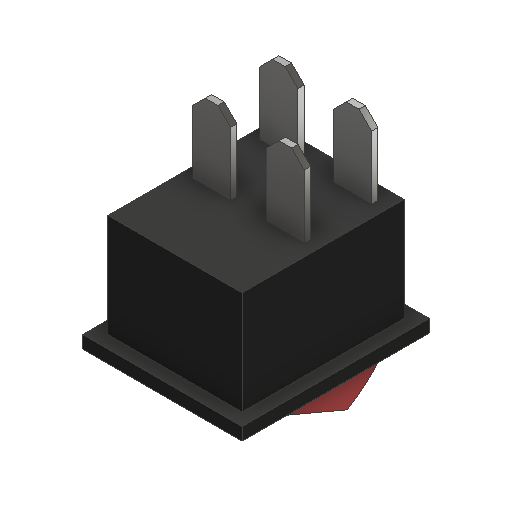
# Autodesk Inventor part: COTS_GENERIC_AC_Power_Switch_10A
Saved by Autodesk Inventor 2026.1 (Build 301233000, 233)
## iProperties
Created: 2016-06-24
Part Number: COTS_GENERIC_AC_Power_Switch_10A
Material: Ogólny
Document SubType Name: Modeling
Designer: Andrzej
Density: 1 g/cm^3
Appearance: Kauczuk - czarny
Mass: 12.2354 g
Surface Area: 41.2399 cm^2
Volume: 12.2354 cm^3
Author: Andrzej
Autodesk Inventor part; units mm, degrees
ref_plane "YZ Plane" through (0, 0, 0) normal (1, 0, 0) x (0, 1, 0)
ref_plane "XZ Plane" through (0, 0, 0) normal (0, 1, 0) x (-1, 0, 0)
sketch "Szkic1" plane through (0, 0, 0) normal (0, 0, 1) x (1, 0, 0)
  line L0 (-7.5735, 20.8135) -> (13.6265, 20.8135)
  line L1 (13.6265, 20.8135) -> (13.6265, -4.7865)
  line L2 (13.6265, -4.7865) -> (-7.5735, -4.7865)
  line L3 (-7.5735, -4.7865) -> (-7.5735, 20.8135)
  line L4 (-9.5735, 22.8135) -> (15.6265, 22.8135)
  line L5 (15.6265, 22.8135) -> (15.6265, -6.7865)
  line L6 (15.6265, -6.7865) -> (-9.5735, -6.7865)
  line L7 (-9.5735, -6.7865) -> (-9.5735, 22.8135)
  point P0 (0, 0)
  dimension "d0" = 21.2
  dimension "d1" = 25.6
  dimension "d2" = 2
  constraints: 16 end point, 4 parallel, 2 perpendicular, 1 horizontal, 3 other
  measures "d0" distance of L1.end L2.end
  measures "d1" distance of L2.end L0.start
  measures "d2" distance between parallel lines of L3 L7
extrude "Wyciągnięcie proste1" add sketch "Szkic1" along normal blind 16.3 contours L0 L1 L2 L3
extrude "Wyciągnięcie proste2" add sketch "Szkic1" against normal blind 2 contours L0 L1 L2 L3 | L4 L5 L6 L7
ref_plane "Płaszczyzna konstrukcyjna1" through (12.6265, -6.7865, 0) normal (1, 0, 0) x (0, 0, -1)
sketch "Szkic2" plane through (12.6265, -6.7865, 0) normal (1, 0, 0) x (0, 0, -1)
  line L0 (2, 0) -> (2, 29.6) projected
  line L1 (0, 0) -> (2, 0) projected
  line L2 (0, 29.6) -> (2, 29.6) projected
  line L3 (0, 27.6) -> (-16.3, 27.6) projected
  line L4 (0, 2) -> (-16.3, 2) projected
  arc A0 (9, 19.6) -> (2, 26.6) centre (-7.5761, 10.0239) ccw
  line L5 (9, 19.6) -> (2, 3)
  point P0 (0, 6.7865)
  dimension "d8" = 7
  dimension "d9" = 29.6
  dimension "d10" = 2
  dimension "d11" = 10
  dimension "d12" = 1
  dimension "d13" = 1
  constraints: 2 end point, 2 point on circle, 2 point on line, 1 centre point
  measures "d8" distance from line of L5.start L0
  measures "d9" distance between parallel lines of L1 L2
  measures "d10" distance between parallel lines of L2 L3
  measures "d11" distance from line of L2 L5.start
  measures "d12" distance from line of L3 A0.end
  measures "d13" distance from line of L4 L5.end
extrude "Wyciągnięcie proste3" add sketch "Szkic2" against normal blind 18.7
sketch "Szkic3" plane through (0, 0, 16.3) normal (0, 0, 1) x (1, 0, 0)
  line L0 (13.6265, 20.8135) -> (-7.5735, 20.8135) projected
  line L1 (-7.5735, 20.8135) -> (-7.5735, -4.7865) projected
  line L2 (-7.5735, -4.7865) -> (13.6265, -4.7865) projected
  line L3 (13.6265, -4.7865) -> (13.6265, 20.8135) projected
  line L4 (-5.9377, 18.5947) -> (0.0623, 18.5947)
  line L5 (0.0623, 18.5947) -> (0.0623, 17.5947)
  line L6 (0.0623, 17.5947) -> (-5.9377, 17.5947)
  line L7 (-5.9377, 17.5947) -> (-5.9377, 18.5947)
  line L8 (5.7192, 18.5947) -> (11.7192, 18.5947)
  line L9 (11.7192, 18.5947) -> (11.7192, 17.5947)
  line L10 (11.7192, 17.5947) -> (5.7192, 17.5947)
  line L11 (5.7192, 17.5947) -> (5.7192, 18.5947)
  line L12 (-5.9377, 7.9577) -> (0.0623, 7.9577)
  line L13 (0.0623, 7.9577) -> (0.0623, 6.9577)
  line L14 (0.0623, 6.9577) -> (-5.9377, 6.9577)
  line L15 (-5.9377, 6.9577) -> (-5.9377, 7.9577)
  line L16 (5.7192, 7.9577) -> (11.7192, 7.9577)
  line L17 (11.7192, 7.9577) -> (11.7192, 6.9577)
  line L18 (11.7192, 6.9577) -> (5.7192, 6.9577)
  line L19 (5.7192, 6.9577) -> (5.7192, 7.9577)
  point P0 (0, 0)
  dimension "d16" = 6
  dimension "d17" = 1
  dimension "d18" = 6
  dimension "d19" = 1
  dimension "d20" = 6
  dimension "d21" = 1
  dimension "d22" = 6
  dimension "d23" = 1
  constraints: 32 end point, 8 parallel, 4 horizontal, 4 perpendicular
  measures "d16" distance of L5.end L6.end
  measures "d17" distance of L4.end L5.end
  measures "d18" distance of L10.start L10.end
  measures "d19" distance of L8.end L10.start
  measures "d20" distance of L14.start L14.end
  measures "d21" distance of L12.end L14.start
  measures "d22" distance of L18.start L18.end
  measures "d23" distance of L16.end L18.start
extrude "Wyciągnięcie proste4" add sketch "Szkic3" along normal blind 12 contours L4 L5 L6 L7 | L8 L9 L10 L11 | L12 L13 L14 L15 | L16 L17 L18 L19
chamfer "Faza1" distance 2 angle 45 8 edges at (0.0623, 18.0947, 28.3) (-5.9377, 18.0947, 28.3) (11.7192, 18.0947, 28.3) (5.7192, 18.0947, 28.3) (11.7192, 7.4577, 28.3) (5.7192, 7.4577, 28.3) (0.0623, 7.4577, 28.3) (-5.9377, 7.4577, 28.3)
sketch "Szkic4" plane through (12.6265, -3.7865, -2) normal (0, -0.3886, -0.9214) x (-1, 0, 0)
  line L0 (6.8473, 17.5297) -> (14.0234, 17.5297) construction
  line L1 (14.0234, 17.5297) -> (14.0234, 9.4771) construction
  line L2 (14.0234, 9.4771) -> (6.8473, 9.4771) construction
  line L3 (6.8473, 9.4771) -> (6.8473, 17.5297) construction
  line L4 (8.3846, 8.6266) -> (9.6316, 8.6266) construction
  line L5 (9.6316, 8.6266) -> (9.6316, 4.3438) construction
  line L6 (9.6316, 4.3438) -> (8.3846, 4.3438) construction
  line L7 (8.3846, 4.3438) -> (8.3846, 8.6266) construction
  constraints: 4 other
